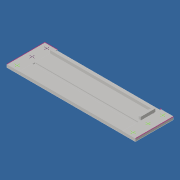
# Autodesk Inventor part: Fixture Base
Saved by Autodesk Inventor 2016 (Build 200138000, 138)
## iProperties
Created: 2016-04-07
Part Number: Fixture Base
Material: Generic
Document SubType Name: Modeling
Designer: Sam Clay
Density: 1 g/cm^3
Appearance: Default
Author: Sam Clay
Autodesk Inventor part; units mm, degrees
ref_plane "YZ Plane" through (0, 0, 0) normal (1, 0, 0) x (0, 1, 0)
ref_plane "XZ Plane" through (0, 0, 0) normal (0, 1, 0) x (-1, 0, 0)
ref_plane "XY Plane" through (0, 0, 0) normal (0, 0, 1) x (1, 0, 0)
sketch "Sketch1" plane through (0, 0, 0) normal (0, 1, 0) x (-1, 0, 0)
  line L0 (0, 0) -> (622.3, 0)
  line L1 (622.3, 0) -> (622.3, 228.6)
  line L2 (622.3, 228.6) -> (0, 228.6)
  line L3 (0, 228.6) -> (0, 0)
  line L4 (0, 228.6) -> (-76.2, 228.6)
  line L5 (-76.2, 228.6) -> (-76.2, 0)
  line L6 (-76.2, 0) -> (0, 0)
  line L7 (0, 0) -> (0, 228.6)
  line L8 (622.3, 228.6) -> (698.5, 228.6)
  line L9 (698.5, 228.6) -> (698.5, 0)
  line L10 (698.5, 0) -> (622.3, 0)
  line L11 (622.3, 0) -> (622.3, 228.6)
  dimension "d0" = 622.3
  dimension "d1" = 228.6
  dimension "d87" = 76.2
  dimension "d88" = 76.2
  constraints: 24 end point, 6 parallel, 3 horizontal, 3 perpendicular, 1 point on line
  measures "d0" distance of L2.end L1.end
  measures "d1" distance of L1.end L0.end
  measures "d87" distance of L6.end L5.end
  measures "d88" distance of L9.end L10.end
extrude "Extrusion1" add sketch "Sketch1" along normal blind 19.05 contours L3 L2 L1 L0
sketch "Sketch2" plane through (0, 19.05, 0) normal (0, 1, 0) x (1, 0, 0)
  line L0 (0, 0) -> (-622.3, 0) projected
  line L1 (-622.3, 0) -> (-622.3, -228.6) projected
  line L2 (0, 0) -> (-622.3, 0)
  line L3 (-622.3, 0) -> (-622.3, -19.05)
  line L4 (-622.3, -19.05) -> (0, -19.05)
  line L5 (0, -19.05) -> (0, 0)
  line L6 (0, 0) -> (-12.7, 0)
  line L7 (-12.7, 0) -> (-12.7, -120.65)
  line L8 (-12.7, -120.65) -> (0, -120.65)
  line L9 (0, -120.65) -> (0, 0)
  line L10 (0, -152.4) -> (-622.3, -152.4)
  line L11 (-622.3, -152.4) -> (-622.3, -133.35)
  line L12 (-622.3, -133.35) -> (0, -133.35)
  line L13 (0, -133.35) -> (0, -152.4)
  line L14 (0, -44.45) -> (-622.3, -44.45)
  line L15 (-622.3, -44.45) -> (-622.3, -31.75)
  line L16 (-622.3, -31.75) -> (0, -31.75)
  line L17 (0, -31.75) -> (0, -44.45)
  line L18 (-12.7, -42.5371) -> (-10.7871, -44.45)
  line L19 (-12.7, -42.5371) -> (-15.4053, -42.5371) construction
  circle A0 centre (-14.2621, -46.0121) radius 3.81
  point P0 (-12.7, -19.05)
  point P1 (-12.7, -44.45)
  point P2 (-12.7, -44.45)
  dimension "d4" = 19.05
  dimension "d5" = 12.7
  dimension "d75" = 19.05
  dimension "d76" = 12.7
  dimension "d77" = 12.7
  dimension "d78" = 12.7
  dimension "d79" = 76.2
  dimension "d83" = 135
  dimension "d84" = 7.62
  constraints: 36 end point, 10 point on line, 8 parallel, 5 horizontal, 4 perpendicular, 2 point on circle, 1 centre point, 1 coincident, 1 equal length
  measures "d4" distance of L3.end L2.end
  measures "d5" distance of L8.end L7.end
  measures "d75" distance of L10.end L11.end
  measures "d76" distance from line of L8.end L12
  measures "d77" distance of L14.end L15.end
  measures "d78" distance between parallel lines of L4 L16
  measures "d79" distance from line of L14 L7.end
  measures "d83" angle of L19 L18
  measures "d84" diameter of A0
extrude "Extrusion2" add sketch "Sketch2" along normal blind 19.05 contours L9 L14 A0 L7 L16 | L7 A0 L14 L1 L16 | L9 L8 L7 A0 L14 | L18 L14 L7 | A0 L18 | L7 L14 A0 | A0 L7 L14 picked at (-15.9132, -44.2053) picked at (-12.45, -47.6591)
extrude "Extrusion9" cut sketch "Sketch2" along normal up to next contours L18 L14 L7 | A0 L18 | L7 L14 A0 | A0 L7 L14 | L7 A0 L14
extrude "Extrusion10" cut sketch "Sketch2" against normal blind 7.62 contours L5 L4 L7 L0 | L7 L4 L1 L0 | L12 L13 L10 L1
extrude "Extrusion11" add sketch "Sketch1" along normal blind 17.78 contours L6 L5 L4 L3 | L1 L8 L9 L10
sketch "Sketch8" plane through (0, 17.78, 0) normal (0, 1, 0) x (1, 0, 0)
  line L0 (-622.3, 0) -> (-698.5, 0) projected
  line L1 (-698.5, 0) -> (-698.5, -228.6) projected
  line L2 (76.2, -228.6) -> (76.2, 0) projected
  point P0 (0, 0)
  point P1 (-660.4, -25.4)
  point P2 (-660.4, -114.3)
  point P3 (-660.4, -203.2)
  point P4 (38.1, -203.2)
  point P5 (38.1, -114.3)
  point P6 (38.1, -25.4)
  dimension "d91" = 25.4
  dimension "d92" = 88.9
  dimension "d93" = 88.9
  dimension "d94" = 38.1
  dimension "d95" = 38.1
  dimension "d96" = 38.1
  constraints: 2 vertical alignment
  measures "d91" distance from line of point (-660.4, -25.4) L0
  measures "d92" distance of point (-660.4, -114.3) point (-660.4, -25.4)
  measures "d93" distance of point (-660.4, -203.2) point (-660.4, -114.3)
  measures "d94" distance from line of L1 point (-660.4, -25.4)
  measures "d95" distance from line of L1 point (-660.4, -114.3)
  measures "d96" distance from line of L2 point (38.1, -203.2)
sketch "Sketch9" plane through (0, 19.05, 0) normal (0, 1, 0) x (1, 0, 0)
  point P0 (0, 0)
  point P1 (-12.7, -44.45)
  point P2 (-12.7, -44.45)
  constraints: 1 coincident
body "Solid1"
